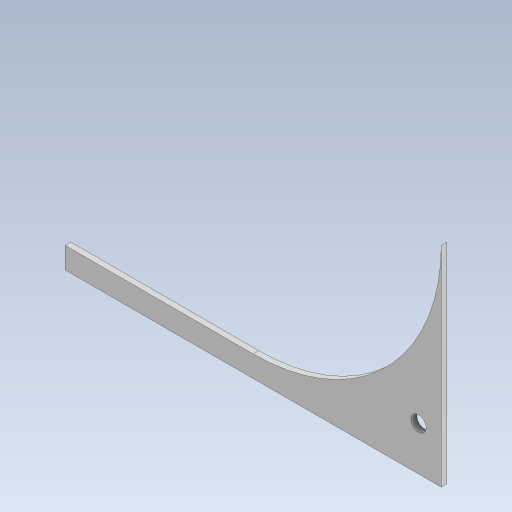
# Autodesk Inventor part: 零件10
Saved by Autodesk Inventor 2023 (Build 270158000, 158)
## iProperties
Created: 2023-05-16
Part Number: 零件10
Material: 一般
Document SubType Name: Modeling
Designer: Johnny Jou
Density: 1 g/cm^3
Appearance: 預設
Author: Johnny Jou
Autodesk Inventor part; units mm, degrees
ref_plane "YZ Plane" through (0, 0, 0) normal (1, 0, 0) x (0, 1, 0)
ref_plane "XZ Plane" through (0, 0, 0) normal (0, 1, 0) x (-1, 0, 0)
ref_plane "XY Plane" through (0, 0, 0) normal (0, 0, 1) x (1, 0, 0)
sketch "草圖1" plane through (0, 0, 0) normal (0, 0, 1) x (1, 0, 0)
  line L0 (0, -80) -> (100, -80)
  arc A0 (100, -80) -> (200, 20) centre (100, 20) ccw
  line L1 (200, 20) -> (200, 40)
  line L2 (200, 40) -> (100, 40)
  line L3 (100, 40) -> (100, -80)
  line L4 (100, -80) -> (200, -80)
  line L5 (200, -80) -> (200, 40)
  line L6 (204.3223, -80) -> (200, -80)
  line L7 (200, -80) -> (200, 40)
  circle A1 centre (188, -68) radius 4
  line L8 (0, -80) -> (200, -80)
  line L9 (200, -80) -> (200, -91.325)
  line L10 (200, -91.325) -> (0, -91.325)
  line L11 (0, -91.325) -> (0, -80)
  line L12 (0, -128.8528) -> (0, 68.1421) projected
  point P0 (200, 20)
  point P1 (200, 20)
  dimension "d6" = 8
  dimension "d7" = 12
  dimension "d8" = 12
  dimension "d9" = 11.325
  constraints: 24 end point, 4 parallel, 3 collinear, 3 horizontal, 2 centre point, 2 perpendicular, 2 point on circle, 1 coincident, 1 vertical, 5 other
  measures "d6" diameter of A1
  measures "d7" distance from line of L5 A1.centre
  measures "d8" distance from line of L4 A1.centre
  measures "d9" distance between parallel lines of L10 L4
extrude "擠出1" add sketch "草圖1" along normal blind 3 contours L0 L4 L9 L10 L11 | A0 L5 L4
